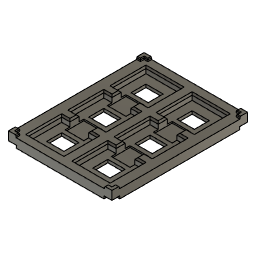
CPU_Tray_LGA_1366 (Autodesk Fusion 360 design; units mm, degrees)
Autodesk Fusion 360 part; units mm, degrees
sketch "Esquisse1" plane through (0, 0, 0) normal (0, 0, 1) x (1, 0, 0)
  line L0 (0, 0) -> (138, 0)
  line L1 (138, 0) -> (138, -181)
  line L2 (138, -181) -> (0, -181)
  line L3 (0, -181) -> (0, 0)
  line L4 (61.6667, -12.25) -> (61.6667, -56.25)
  line L5 (61.6667, -56.25) -> (14.6667, -56.25)
  line L6 (14.6667, -56.25) -> (14.6667, -12.25)
  line L7 (14.6667, -12.25) -> (61.6667, -12.25)
  line L8 (123.3333, -12.25) -> (123.3333, -56.25)
  line L9 (76.3333, -56.25) -> (76.3333, -12.25)
  line L10 (76.3333, -12.25) -> (123.3333, -12.25)
  line L11 (123.3333, -56.25) -> (76.3333, -56.25)
  line L12 (14.6667, -68.5) -> (61.6667, -68.5)
  line L13 (14.6667, -112.5) -> (14.6667, -68.5)
  line L14 (61.6667, -112.5) -> (14.6667, -112.5)
  line L15 (61.6667, -68.5) -> (61.6667, -112.5)
  line L16 (76.3333, -68.5) -> (123.3333, -68.5)
  line L17 (123.3333, -68.5) -> (123.3333, -112.5)
  line L18 (76.3333, -112.5) -> (76.3333, -68.5)
  line L19 (123.3333, -112.5) -> (76.3333, -112.5)
  line L20 (14.6667, -124.75) -> (61.6667, -124.75)
  line L21 (14.6667, -168.75) -> (14.6667, -124.75)
  line L22 (61.6667, -168.75) -> (14.6667, -168.75)
  line L23 (61.6667, -124.75) -> (61.6667, -168.75)
  line L24 (76.3333, -124.75) -> (123.3333, -124.75)
  line L25 (123.3333, -124.75) -> (123.3333, -168.75)
  line L26 (76.3333, -168.75) -> (76.3333, -124.75)
  line L27 (123.3333, -168.75) -> (76.3333, -168.75)
  dimension "d1" = 138
  dimension "d2" = 181
  dimension "d3" = 44
  dimension "d4" = 47
  dimension "d5" = 44
  dimension "d6" = 47
  dimension "d7" = 12.25
  dimension "d8" = 14.6667
  dimension "d9" = 12.25
  dimension "d10" = 14.6667
  dimension "d11" = 44
  dimension "d12" = 47
  dimension "d13" = 44
  dimension "d14" = 47
  dimension "d15" = 44
  dimension "d16" = 47
  dimension "d17" = 44
  dimension "d18" = 47
  dimension "d19" = 14.6667
  dimension "d20" = 14.6667
  dimension "d21" = 14.6667
  dimension "d22" = 14.6667
  dimension "d23" = 12.25
  dimension "d24" = 12.25
  dimension "d25" = 12.25
  dimension "d26" = 12.25
  constraint horizontal L0
  constraint vertical L1
  constraint horizontal L2
  constraint vertical L3
  constraint coincident L0.start L3.end
  measures "d1" distance of L1 L3
  measures "d2" distance of L0 L2
  measures "d3" distance of L5 L7
  measures "d4" distance of L4 L6
  measures "d5" distance of L10 L11
  measures "d6" distance of L8 L9
  measures "d7" distance of L0 L7
  measures "d8" distance of L3 L6
  measures "d9" distance of L0 L10
  measures "d10" distance of L1 L8
  measures "d11" distance of L12 L14
  measures "d12" distance of L13 L15
  measures "d13" distance of L16 L19
  measures "d14" distance of L17 L18
  measures "d15" distance of L20 L22
  measures "d16" distance of L21 L23
  measures "d17" distance of L24 L27
  measures "d18" distance of L25 L26
  measures "d19" distance of L3 L13
  measures "d20" distance of L3 L21
  measures "d21" distance of L1 L17
  measures "d22" distance of L1 L25
  measures "d23" distance of L11 L16
  measures "d24" distance of L19 L24
  measures "d25" distance of L14 L20
  measures "d26" distance of L5 L12
extrude "Extrusion1" add sketch "Esquisse1" along normal blind 4 contours L4 L5 L6 L7 | L8 L9 L10 L11 | L12 L13 L14 L15 | L16 L17 L18 L19 | L20 L21 L22 L23 | L24 L25 L26 L27 makes body 1 at (46, -97.8333, 0) makes body 2 at (46, -26.9167, 0) makes body 3 at (30.3333, -154.0833, 0) makes body 4 at (107.6667, -97.8333, 0) makes body 5 at (107.6667, -41.5833, 0) makes body 6 at (107.6667, -154.0833, 0)
extrude "Extrusion2" add sketch "Esquisse1" along normal blind 10 bodies 1 2 3 4 5 6
sketch "Esquisse2" plane through (0, 0, 0) normal (0, 0, 1) x (1, 0, 0)
  line L0 (0, 0) -> (138, 0)
  line L1 (138, -181) -> (0, -181)
  line L2 (0, -181) -> (0, 0)
  line L3 (138, 0) -> (138, -181)
  line L4 (14.6667, -12.25) -> (61.6667, -12.25)
  line L5 (61.6667, -56.25) -> (14.6667, -56.25)
  line L6 (14.6667, -56.25) -> (14.6667, -12.25)
  line L7 (61.6667, -12.25) -> (61.6667, -56.25)
  line L8 (26.6667, -24.25) -> (49.6667, -24.25)
  line L9 (49.6667, -24.25) -> (49.6667, -44.25)
  line L10 (49.6667, -44.25) -> (26.6667, -44.25)
  line L11 (26.6667, -44.25) -> (26.6667, -24.25)
  line L12 (69, 0) -> (69, -181)
  line L13 (26.6667, -80.5) -> (49.6667, -80.5)
  line L14 (49.6667, -80.5) -> (49.6667, -100.5)
  line L15 (49.6667, -100.5) -> (26.6667, -100.5)
  line L16 (26.6667, -100.5) -> (26.6667, -80.5)
  line L17 (26.6667, -136.75) -> (49.6667, -136.75)
  line L18 (49.6667, -136.75) -> (49.6667, -156.75)
  line L19 (49.6667, -156.75) -> (26.6667, -156.75)
  line L20 (26.6667, -156.75) -> (26.6667, -136.75)
  line L21 (14.6667, -68.5) -> (61.6667, -68.5)
  line L22 (14.6667, -112.5) -> (14.6667, -68.5)
  line L23 (61.6667, -112.5) -> (14.6667, -112.5)
  line L24 (61.6667, -68.5) -> (61.6667, -112.5)
  line L25 (14.6667, -124.75) -> (61.6667, -124.75)
  line L26 (14.6667, -168.75) -> (14.6667, -124.75)
  line L27 (61.6667, -168.75) -> (14.6667, -168.75)
  line L28 (61.6667, -124.75) -> (61.6667, -168.75)
  line L29 (111.3333, -24.25) -> (88.3333, -24.25)
  line L30 (111.3333, -44.25) -> (111.3333, -24.25)
  line L31 (88.3333, -44.25) -> (111.3333, -44.25)
  line L32 (88.3333, -24.25) -> (88.3333, -44.25)
  line L33 (111.3333, -80.5) -> (88.3333, -80.5)
  line L34 (111.3333, -100.5) -> (111.3333, -80.5)
  line L35 (88.3333, -100.5) -> (111.3333, -100.5)
  line L36 (88.3333, -80.5) -> (88.3333, -100.5)
  line L37 (111.3333, -136.75) -> (88.3333, -136.75)
  line L38 (111.3333, -156.75) -> (111.3333, -136.75)
  line L39 (88.3333, -156.75) -> (111.3333, -156.75)
  line L40 (88.3333, -136.75) -> (88.3333, -156.75)
  dimension "d37" = 12
  dimension "d38" = 12
  dimension "d39" = 12
  dimension "d40" = 12
  dimension "d41" = 12
  dimension "d42" = 12
  dimension "d43" = 12
  dimension "d44" = 12
  dimension "d45" = 12
  dimension "d46" = 12
  dimension "d47" = 12
  dimension "d48" = 12
  constraint horizontal L8
  constraint vertical L9
  constraint horizontal L10
  constraint vertical L11
  constraint midpoint L0 L12.start
  constraint midpoint L1 L12.end
  constraint horizontal L13
  constraint vertical L14
  constraint horizontal L15
  constraint vertical L16
  constraint horizontal L17
  constraint vertical L18
  constraint horizontal L19
  constraint vertical L20
  constraint symmetric L8.start L12 L29.start
  constraint symmetric L8.end L12 L29.end
  constraint symmetric L9.end L12 L31.start
  constraint symmetric L10.end L12 L30.start
  constraint symmetric L12 L13.start L33.start
  constraint symmetric L12 L13.end L33.end
  constraint symmetric L12 L14.end L35.start
  constraint symmetric L12 L15.end L34.start
  constraint symmetric L12 L17.start L37.start
  constraint symmetric L12 L17.end L37.end
  constraint symmetric L12 L18.end L39.start
  constraint symmetric L12 L19.end L38.start
  measures "d37" distance of L7 L9
  measures "d38" distance of L6 L11
  measures "d39" distance of L5 L10
  measures "d40" distance of L4 L8
  measures "d41" distance of L13 L21
  measures "d42" distance of L16 L22
  measures "d43" distance of L15 L23
  measures "d44" distance of L14 L24
  measures "d45" distance of L17 L25
  measures "d46" distance of L20 L26
  measures "d47" distance of L19 L27
  measures "d48" distance of L18 L28
extrude "Extrusion3" add 1 faces at (4.8889, -97.8333, 10) along direction (0, 0, 1) blind 2 on bodies 1 bodies 1
extrude "Extrusion4" cut sketch "Esquisse2" along normal blind 5 contours L8 L9 L10 L11 bodies 1
extrude "Extrusion5" cut sketch "Esquisse2" along normal blind 5 contours L13 L14 L15 L16 | L17 L18 L19 L20 | L29 L30 L31 L32 | L33 L34 L35 L36 | L37 L38 L39 L40 bodies 1
sketch "Esquisse3" plane through (0, 0, 0) normal (0, 0, 1) x (1, 0, 0)
  line L0 (5.25, -5.25) -> (10.5, -5.25)
  line L1 (5.25, -10.5) -> (0, -10.5)
  line L2 (10.5, -5.25) -> (10.5, 0)
  line L3 (0.1008, 0) -> (10.5, 0)
  line L4 (5.25, -10.5) -> (5.25, -5.25)
  line L5 (0, -0.1279) -> (0, -10.5)
  line L6 (0, 0) -> (0, -181)
  line L7 (0, 0) -> (138, 0)
  line L8 (69, -0.1066) -> (69, -181)
  line L9 (0, -181) -> (0, 0)
  line L10 (138, 0) -> (138, -181)
  line L11 (0, -90.5) -> (138, -90.5)
  line L12 (138, -181) -> (0, -181)
  line L13 (127.5, -5.25) -> (127.5, 0)
  line L14 (137.8992, 0) -> (127.5, 0)
  line L15 (138, -0.1279) -> (138, -10.5)
  line L16 (132.75, -10.5) -> (138, -10.5)
  line L17 (132.75, -10.5) -> (132.75, -5.25)
  line L18 (132.75, -5.25) -> (127.5, -5.25)
  line L19 (10.5, -175.75) -> (10.5, -181)
  line L20 (0.1008, -181) -> (10.5, -181)
  line L21 (0, -180.8721) -> (0, -170.5)
  line L22 (5.25, -170.5) -> (0, -170.5)
  line L23 (5.25, -175.75) -> (10.5, -175.75)
  line L24 (5.25, -170.5) -> (5.25, -175.75)
  line L25 (127.5, -175.75) -> (127.5, -181)
  line L26 (137.8992, -181) -> (127.5, -181)
  line L27 (138, -180.8721) -> (138, -170.5)
  line L28 (132.75, -175.75) -> (127.5, -175.75)
  line L29 (132.75, -170.5) -> (132.75, -175.75)
  line L30 (132.75, -170.5) -> (138, -170.5)
  point P0 (0, -0.1279)
  point P1 (0, -0.1066)
  point P2 (69, -0.1066)
  dimension "d67" = 10.5
  dimension "d68" = 10.5
  dimension "d69" = 5.25
  dimension "d70" = 5.25
  dimension "d71" = 69
  dimension "d72" = 138
  dimension "d73" = 181
  dimension "d74" = 90.5
  constraint collinear L5 L6
  constraint collinear L3 L7
  constraint coincident P2 L8.start
  constraint perpendicular L7 L8
  constraint coincident L6 L11.start
  constraint coincident L10 L11.end
  constraint perpendicular L10 L11
  constraint symmetric P0 L8 L15.start
  constraint symmetric L1.start L8 L16.start
  constraint symmetric L2.end L8 L13.end
  constraint symmetric L0.end L8 L13.start
  constraint symmetric L1.end L8 L15.end
  constraint symmetric L0.start L8 L17.end
  constraint symmetric L3.start L8 L14.start
  constraint symmetric P0 L11 L21.start
  constraint symmetric L1.start L11 L22.start
  constraint symmetric L2.end L11 L19.end
  constraint symmetric L0.end L11 L19.start
  constraint symmetric L1.end L11 L21.end
  constraint symmetric L0.start L11 L23.start
  constraint symmetric L3.start L11 L20.start
  constraint symmetric L11 L13.start L25.start
  constraint symmetric L11 L13.end L25.end
  constraint symmetric L11 L14.start L26.start
  constraint symmetric L11 L15.start L27.start
  constraint symmetric L11 L15.end L27.end
  constraint symmetric L11 L16.start L29.start
  constraint symmetric L11 L17.end L28.start
  measures "d67" distance of L2 L5
  measures "d68" distance of L1 L3
  measures "d69" distance of L2 L4
  measures "d70" distance of L1.start L0.start
  measures "d71" distance of L8 L9
  measures "d72" distance of L9 L10
  measures "d73" distance of L7 L12
  measures "d74" distance of L7 L11
extrude "Extrusion8" cut sketch "Esquisse3" along normal blind 3.5 contours L0 L1 L2 L3 L4 L5 L6 L7 L9 | L7 L10 L13 L14 L15 L16 L17 L18 | L6 L9 L12 L19 L20 L21 L22 L23 L24 | L10 L12 L25 L26 L27 L28 L29 L30 bodies 1
sketch "Esquisse4" plane through (0, 0, 12) normal (0, 0, 1) x (-1, 0, 0)
  line L0 (-14.6667, 56.25) -> (-14.6667, 12.25)
  line L1 (-14.6667, 12.25) -> (-61.6667, 12.25)
  line L2 (-61.6667, 12.25) -> (-61.6667, 56.25)
  line L3 (-61.6667, 56.25) -> (-14.6667, 56.25)
  line L4 (-123.3333, 12.25) -> (-123.3333, 56.25)
  line L5 (-123.3333, 56.25) -> (-76.3333, 56.25)
  line L6 (-76.3333, 56.25) -> (-76.3333, 12.25)
  line L7 (-76.3333, 12.25) -> (-123.3333, 12.25)
  line L8 (-14.6667, 68.5) -> (-61.6667, 68.5)
  line L9 (-61.6667, 68.5) -> (-61.6667, 112.5)
  line L10 (-61.6667, 112.5) -> (-14.6667, 112.5)
  line L11 (-14.6667, 112.5) -> (-14.6667, 68.5)
  line L12 (-123.3333, 68.5) -> (-123.3333, 112.5)
  line L13 (-123.3333, 112.5) -> (-76.3333, 112.5)
  line L14 (-76.3333, 112.5) -> (-76.3333, 68.5)
  line L15 (-76.3333, 68.5) -> (-123.3333, 68.5)
  line L16 (-14.6667, 124.75) -> (-61.6667, 124.75)
  line L17 (-61.6667, 124.75) -> (-61.6667, 168.75)
  line L18 (-61.6667, 168.75) -> (-14.6667, 168.75)
  line L19 (-14.6667, 168.75) -> (-14.6667, 124.75)
  line L20 (-123.3333, 124.75) -> (-123.3333, 168.75)
  line L21 (-123.3333, 168.75) -> (-76.3333, 168.75)
  line L22 (-76.3333, 168.75) -> (-76.3333, 124.75)
  line L23 (-76.3333, 124.75) -> (-123.3333, 124.75)
  line L24 (0, 181) -> (-138, 181)
  line L25 (-138, 181) -> (-138, 0)
  line L26 (-138, 0) -> (0, 0)
  line L27 (0, 0) -> (0, 181)
  line L28 (-25.6667, 49.875) -> (-50.6667, 49.875)
  line L29 (-50.6667, 49.875) -> (-50.6667, 74.875)
  line L30 (-50.6667, 74.875) -> (-25.6667, 74.875)
  line L31 (-25.6667, 74.875) -> (-25.6667, 49.875)
  line L32 (-69, 0) -> (-69, 181)
  line L33 (-25.6667, 106.125) -> (-50.6667, 106.125)
  line L34 (-50.6667, 106.125) -> (-50.6667, 131.125)
  line L35 (-50.6667, 131.125) -> (-25.6667, 131.125)
  line L36 (-25.6667, 131.125) -> (-25.6667, 106.125)
  line L37 (-112.3333, 49.875) -> (-87.3333, 49.875)
  line L38 (-112.3333, 74.875) -> (-112.3333, 49.875)
  line L39 (-87.3333, 74.875) -> (-112.3333, 74.875)
  line L40 (-87.3333, 49.875) -> (-87.3333, 74.875)
  line L41 (-112.3333, 106.125) -> (-87.3333, 106.125)
  line L42 (-112.3333, 131.125) -> (-112.3333, 106.125)
  line L43 (-87.3333, 131.125) -> (-112.3333, 131.125)
  line L44 (-87.3333, 106.125) -> (-87.3333, 131.125)
  dimension "d55" = 25
  dimension "d56" = 25
  dimension "d57" = 6.375
  dimension "d58" = 12.25
  dimension "d59" = 11
  dimension "d60" = 47
  dimension "d61" = 25
  dimension "d62" = 25
  dimension "d63" = 6.375
  dimension "d64" = 11
  constraint horizontal L28
  constraint vertical L29
  constraint horizontal L30
  constraint vertical L31
  constraint midpoint L26 L32.start
  constraint midpoint L24 L32.end
  constraint horizontal L33
  constraint vertical L34
  constraint horizontal L35
  constraint vertical L36
  constraint symmetric L28.start L32 L37.start
  constraint symmetric L28.end L32 L37.end
  constraint symmetric L29.end L32 L39.start
  constraint symmetric L30.end L32 L38.start
  constraint symmetric L32 L33.start L41.start
  constraint symmetric L32 L33.end L41.end
  constraint symmetric L32 L34.end L43.start
  constraint symmetric L32 L35.end L42.start
  measures "d55" distance of L28 L30
  measures "d56" distance of L29 L31
  measures "d57" distance of L3 L28
  measures "d58" distance of L3 L8
  measures "d59" distance of L0 L31
  measures "d60" distance of L0 L2
  measures "d61" distance of L33 L35
  measures "d62" distance of L34 L36
  measures "d63" distance of L10 L33
  measures "d64" distance of L11 L36
extrude "Extrusion7" cut sketch "Esquisse4" against normal blind 10 contours L3 L28 L29 L31 | L3 L8 L29 L31 | L8 L29 L30 L31 | L10 L33 L34 L36 | L10 L16 L34 L36 | L16 L34 L35 L36 | L5 L15 L38 L40 | L5 L37 L38 L40 | L15 L38 L39 L40 | L13 L23 L42 L44 | L13 L41 L42 L44 | L23 L42 L43 L44 bodies 1
sketch "Esquisse5" plane through (0, 0, 12) normal (0, 0, 1) x (-1, 0, 0)
  line L0 (-112.3333, 56.25) -> (-112.3333, 68.5)
  line L1 (-112.3333, 68.5) -> (-123.3333, 68.5)
  line L2 (-123.3333, 68.5) -> (-123.3333, 112.5)
  line L3 (-123.3333, 112.5) -> (-112.3333, 112.5)
  line L4 (-112.3333, 112.5) -> (-112.3333, 124.75)
  line L5 (-112.3333, 124.75) -> (-123.3333, 124.75)
  line L6 (-123.3333, 124.75) -> (-123.3333, 168.75)
  line L7 (-123.3333, 168.75) -> (-76.3333, 168.75)
  line L8 (-76.3333, 168.75) -> (-76.3333, 124.75)
  line L9 (-76.3333, 124.75) -> (-87.3333, 124.75)
  line L10 (-87.3333, 124.75) -> (-87.3333, 112.5)
  line L11 (-87.3333, 112.5) -> (-76.3333, 112.5)
  line L12 (-76.3333, 112.5) -> (-76.3333, 68.5)
  line L13 (-76.3333, 68.5) -> (-87.3333, 68.5)
  line L14 (-87.3333, 68.5) -> (-87.3333, 56.25)
  line L15 (-87.3333, 56.25) -> (-76.3333, 56.25)
  line L16 (-76.3333, 56.25) -> (-76.3333, 12.25)
  line L17 (-76.3333, 12.25) -> (-123.3333, 12.25)
  line L18 (-123.3333, 12.25) -> (-123.3333, 56.25)
  line L19 (-123.3333, 56.25) -> (-112.3333, 56.25)
  line L20 (-50.6667, 56.25) -> (-50.6667, 68.5)
  line L21 (-50.6667, 68.5) -> (-61.6667, 68.5)
  line L22 (-61.6667, 68.5) -> (-61.6667, 112.5)
  line L23 (-61.6667, 112.5) -> (-50.6667, 112.5)
  line L24 (-50.6667, 112.5) -> (-50.6667, 124.75)
  line L25 (-50.6667, 124.75) -> (-61.6667, 124.75)
  line L26 (-61.6667, 124.75) -> (-61.6667, 168.75)
  line L27 (-61.6667, 168.75) -> (-14.6667, 168.75)
  line L28 (-14.6667, 168.75) -> (-14.6667, 124.75)
  line L29 (-14.6667, 124.75) -> (-25.6667, 124.75)
  line L30 (-25.6667, 124.75) -> (-25.6667, 112.5)
  line L31 (-25.6667, 112.5) -> (-14.6667, 112.5)
  line L32 (-14.6667, 112.5) -> (-14.6667, 68.5)
  line L33 (-14.6667, 68.5) -> (-25.6667, 68.5)
  line L34 (-25.6667, 68.5) -> (-25.6667, 56.25)
  line L35 (-25.6667, 56.25) -> (-14.6667, 56.25)
  line L36 (-14.6667, 56.25) -> (-14.6667, 12.25)
  line L37 (-14.6667, 12.25) -> (-61.6667, 12.25)
  line L38 (-61.6667, 12.25) -> (-61.6667, 56.25)
  line L39 (-61.6667, 56.25) -> (-50.6667, 56.25)
  line L40 (0, 181) -> (-138, 181)
  line L41 (-138, 181) -> (-138, 0)
  line L42 (-138, 0) -> (0, 0)
  line L43 (0, 0) -> (0, 181)
  line L44 (0, 0) -> (-10, 0)
  line L45 (-10, 5) -> (-5, 5)
  line L46 (-5, 5) -> (-5, 10)
  line L47 (-5, 10) -> (0, 10)
  line L48 (0, 0) -> (0, 10)
  line L49 (-10, 0) -> (-10, 5)
  line L50 (-69, 0) -> (-69, 181)
  line L51 (0, 90.5) -> (-138, 90.5)
  line L52 (-138, 0) -> (-138, 10)
  line L53 (-133, 5) -> (-133, 10)
  line L54 (-128, 5) -> (-133, 5)
  line L55 (-128, 0) -> (-128, 5)
  line L56 (-138, 0) -> (-128, 0)
  line L57 (-133, 10) -> (-138, 10)
  line L58 (0, 181) -> (0, 171)
  line L59 (0, 181) -> (-10, 181)
  line L60 (-10, 181) -> (-10, 176)
  line L61 (-10, 176) -> (-5, 176)
  line L62 (-5, 176) -> (-5, 171)
  line L63 (-5, 171) -> (0, 171)
  line L64 (-128, 181) -> (-128, 176)
  line L65 (-138, 181) -> (-128, 181)
  line L66 (-138, 181) -> (-138, 171)
  line L67 (-133, 171) -> (-138, 171)
  line L68 (-133, 176) -> (-133, 171)
  line L69 (-128, 176) -> (-133, 176)
  point P0 (-138, 0)
  constraint coincident L42.end L43.start
  constraint coincident L42 L44.end
  constraint perpendicular L43 L44
  constraint perpendicular L43 L45
  constraint perpendicular L45 L46
  constraint perpendicular L46 L47
  constraint perpendicular L47 L48
  constraint perpendicular L45 L49
  constraint midpoint L42 L50.start
  constraint midpoint L40 L50.end
  constraint midpoint L43 L51.start
  constraint midpoint L41 L51.end
  constraint symmetric L42.end L50 L41.end
  constraint symmetric L42.end L50 P0
  constraint symmetric L44.end L50 L55.start
  constraint symmetric L45.start L50 L54.start
  constraint symmetric L45.end L50 L53.start
  constraint symmetric L46.end L50 L53.end
  constraint symmetric L47.end L50 L52.end
  constraint symmetric L42.end L51 L40.start
  constraint symmetric L44.end L51 L59.end
  constraint symmetric L45.start L51 L60.end
  constraint symmetric L45.end L51 L61.end
  constraint symmetric L46.end L51 L62.end
  constraint symmetric L47.end L51 L58.end
  constraint symmetric L51 L55.start L64.start
  constraint symmetric L51 P0 L40.end
  constraint symmetric L51 L52.end L66.end
  constraint symmetric L51 L53.start L68.start
  constraint symmetric L51 L53.end L67.start
  constraint symmetric L51 L54.start L64.end
extrude "Extrusion9" add sketch "Esquisse5" along normal blind 3 contours L40 L41 L64 L65 L66 L67 L68 L69 | L41 L42 L52 L53 L54 L55 L56 L57 | L42 L43 L44 L45 L46 L47 L48 L49 | L40 L43 L58 L59 L60 L61 L62 L63 bodies 1
chamfer "Chanfrein1" distance 1 angle 45 16 edges at (128, -2.5, 15) (130.5, -5, 15) (133, -7.5, 15) (135.5, -10, 15) (128, -178.5, 15) (130.5, -176, 15) (133, -173.5, 15) (135.5, -171, 15) (2.5, -171, 15) (5, -173.5, 15) (7.5, -176, 15) (10, -178.5, 15) (2.5, -10, 15) (5, -7.5, 15) (7.5, -5, 15) (10, -2.5, 15) on bodies 1
chamfer "Chanfrein2" distance 2 angle 45 40 edges at (14.6667, -34.25, 12) (61.6667, -34.25, 12) (56.1667, -56.25, 12) (50.6667, -62.375, 12) (56.1667, -68.5, 12) (61.6667, -90.5, 12) (25.6667, -62.375, 12) (20.1667, -56.25, 12) (38.1667, -12.25, 12) (20.1667, -68.5, 12) (14.6667, -90.5, 12) (20.1667, -112.5, 12) (25.6667, -118.625, 12) (20.1667, -124.75, 12) (14.6667, -146.75, 12) (38.1667, -168.75, 12) (61.6667, -146.75, 12) (56.1667, -124.75, 12) (50.6667, -118.625, 12) (56.1667, -112.5, 12) (76.3333, -90.5, 12) (87.3333, -118.625, 12) (81.8333, -112.5, 12) (81.8333, -124.75, 12) (76.3333, -146.75, 12) (99.8333, -168.75, 12) (123.3333, -146.75, 12) (117.8333, -124.75, 12) (112.3333, -118.625, 12) (117.8333, -112.5, 12) (123.3333, -90.5, 12) (117.8333, -68.5, 12) (112.3333, -62.375, 12) (117.8333, -56.25, 12) (123.3333, -34.25, 12) (99.8333, -12.25, 12) (76.3333, -34.25, 12) (81.8333, -56.25, 12) (87.3333, -62.375, 12) (81.8333, -68.5, 12) on bodies 1
equation "d7 = ( d2 - ( 3 * d3 ) ) / 4"
equation "d8 = ( d1 - ( 2 * d4 ) ) / 3"
equation "d9 = d7"
equation "d10 = d8"
equation "d21 = d8"
equation "d23 = d9"
equation "d24 = d23"
equation "d25 = d7"
equation "d26 = d7"
equation "d57 = ( d55 - d58 ) / 2"
equation "d59 = ( d60 - d56 ) / 2"
equation "d61 = d55"
equation "d62 = d56"
equation "d63 = d57"
equation "d64 = d59"
equation "d71 = d72 / 2"
equation "d74 = d73 / 2"
